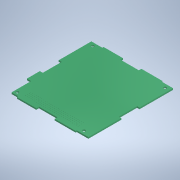
# Autodesk Inventor part: PC104Plus
Saved by Autodesk Inventor 2022 (Build 260153000, 153)
## iProperties
Created: 2021-10-06
Part Number: PC104Plus
Material: Generic
Document SubType Name: Modeling
Designer: Bowen O'Steen
Density: 1 g/cm^3
Appearance: Smooth - Dark Sea Green
Author: Bowen O'Steen
Autodesk Inventor part; units mm, degrees
ref_plane "YZ Plane" through (0, 0, 0) normal (1, 0, 0) x (0, 1, 0)
ref_plane "XZ Plane" through (0, 0, 0) normal (0, 1, 0) x (-1, 0, 0)
ref_plane "XY Plane" through (0, 0, 0) normal (0, 0, 1) x (1, 0, 0)
sketch "Sketch1" plane through (0, 0, 0) normal (0, 1, 0) x (-1, 0, 0)
  line L0 (-23.72, 8.26) -> (89.65, 8.26)
  line L1 (89.65, 8.26) -> (89.65, -95.8987)
  line L2 (89.65, -95.8987) -> (-23.72, -95.8987)
  line L3 (-23.72, -95.8987) -> (-23.72, 8.26)
  line L4 (73.66, 0) -> (0, 0) construction
  line L5 (76.2, -85.73) -> (-3.81, -85.73) construction
  line L6 (4.0755, 3.8152) -> (-8.73, 3.8152)
  line L7 (-8.73, 3.8152) -> (-8.73, -32.5844)
  line L8 (-8.73, -32.5844) -> (-5.9617, -32.5844)
  line L9 (-5.9617, -32.5844) -> (-5.9617, -52.7158)
  line L10 (-5.9617, -52.7158) -> (-8.73, -52.7158)
  line L11 (-8.73, -52.7158) -> (-8.73, -89.8581)
  line L12 (-8.73, -89.8581) -> (4.0755, -89.8581)
  line L13 (4.0755, -89.8581) -> (4.0755, -90.9268)
  line L14 (4.0755, -90.9268) -> (27.3569, -90.9268)
  line L15 (27.3569, -90.9268) -> (27.3569, -88.0825)
  line L16 (27.3569, -88.0825) -> (47.7655, -88.0825)
  line L17 (47.7655, -88.0825) -> (47.7655, -90.9268)
  line L18 (47.7655, -90.9268) -> (69.1789, -90.9268)
  line L19 (69.1789, -90.9268) -> (69.1789, -89.5046)
  line L20 (69.1789, -89.5046) -> (81.2966, -89.5046)
  line L21 (4.0755, 3.8152) -> (4.0755, 4.9196)
  line L22 (4.0755, 4.9196) -> (27.3569, 4.9196)
  line L23 (27.3569, 4.9196) -> (27.3569, 1.943)
  line L24 (27.3569, 1.943) -> (47.7655, 1.943)
  line L25 (47.7655, 1.943) -> (47.7655, 4.9196)
  line L26 (47.7655, 4.9196) -> (69.1789, 4.9196)
  line L27 (69.1789, 4.9196) -> (69.1789, 3.4313)
  line L28 (69.1789, 3.4313) -> (76.6144, 3.4313)
  line L29 (76.6144, 3.4313) -> (76.6144, -18.2014)
  line L30 (76.6144, -18.2014) -> (81.2966, -18.2014)
  line L31 (81.2966, -18.2014) -> (81.2966, -32.5844)
  line L32 (81.2966, -32.5844) -> (78.0605, -32.5844)
  line L33 (78.0605, -32.5844) -> (78.0605, -53.5084)
  line L34 (78.0605, -53.5084) -> (81.2966, -53.5084)
  line L35 (81.2966, -53.5084) -> (81.2966, -89.5046)
  circle A0 centre (73.66, 0) radius 1.59
  circle A1 centre (76.2, -85.73) radius 1.59
  circle A2 centre (-3.81, -85.73) radius 1.59
  circle A3 centre (0, 0) radius 1.59
  dimension "d1" = 73.66
  dimension "d5" = 80.01
  dimension "d6" = 113.37
  dimension "d8" = 15.99
  dimension "d10" = 23.72
  dimension "d11" = 8.26
  dimension "d13" = 85.73
  dimension "d16" = 2.54
  dimension "d52" = 3.18
  dimension "d53" = 3.18
  dimension "d54" = 3.18
  dimension "d55" = 3.18
  constraints: 64 end point, 24 perpendicular, 7 point on line, 5 coincident, 4 centre point, 3 horizontal, 2 vertical, 2 other
  measures "d1" distance of L4.end L4.start
  measures "d5" distance of L5.end L5.start
  measures "d6" distance of L0.start L0.end
  measures "d8" distance from line of L1 L4.start
  measures "d10" distance from line of L3 L4.end
  measures "d11" distance from line of L0 L4.start
  measures "d13" distance between parallel lines of L5 L4
  measures "d16" horizontal distance of L5.start L4.start
  measures "d52" diameter of A0
  measures "d53" diameter of A1
  measures "d54" diameter of A2
  measures "d55" diameter of A3
extrude "Extrusion1" add sketch "Sketch1" along normal blind 1.57 contours L21 L22 L23 L24 L25 L26 L27 L28 L29 L30 L31 L32 L33 L34 L35 L20 L19 L18 L17 L16 L15 L14 L13 L12 L11 L10 L9 L8 L7 L6
sketch "Sketch2" plane through (0, 1.57, 0) normal (0, 1, 0) x (1, 0, 0)
  line L0 (-7.87, 1.24) -> (-7.37, 1.24)
  line L1 (-7.37, 1.24) -> (-7.37, 0.74)
  line L2 (-7.37, 0.74) -> (-7.87, 0.74)
  line L3 (-7.87, 0.74) -> (-7.87, 1.24)
  point P0 (0, 0)
  point P1 (-7.62, 0.99)
  point P2 (-7.37, 0.99)
  point P3 (-7.62, 1.24)
  dimension "d58" = 0.99
  dimension "d59" = 7.62
  dimension "d60" = 0.5
  dimension "d61" = 0.5
  constraints: 8 end point, 2 midpoint, 2 parallel, 1 horizontal, 1 horizontal alignment, 1 perpendicular, 1 vertical alignment
  measures "d58" vertical distance of point (0, 0) point (-7.62, 0.99)
  measures "d59" horizontal distance of point (0, 0) point (-7.62, 0.99)
  measures "d60" distance of L0.end L1.end
  measures "d61" distance of L0.start L0.end
extrude "Extrusion2" cut sketch "Sketch2" against normal through all
pattern_linear "Rectangular Pattern1" count 30 spacing 2 along (-1, 0, 0) count 4 spacing 2 along (0, 0, -1) of "Extrusion2"
body "Solid1"
